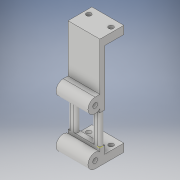
# Autodesk Inventor part: zaxis_clamp2
Saved by Autodesk Inventor 2019 (Build 230136000, 136)
## iProperties
Created: 2020-02-02
Material: Generic
Document SubType Name: Modeling
Designer: Nishant
Density: 1 g/cm^3
Appearance: Default
Author: Nishant
Autodesk Inventor part; units mm, degrees
ref_plane "YZ Plane" through (0, 0, 0) normal (1, 0, 0) x (0, 1, 0)
ref_plane "XZ Plane" through (0, 0, 0) normal (0, 1, 0) x (-1, 0, 0)
ref_plane "XY Plane" through (0, 0, 0) normal (0, 0, 1) x (1, 0, 0)
sketch "Sketch1" plane through (0, 0, 0) normal (1, 0, 0) x (0, 1, 0)
  line L0 (40, 0) -> (40, 3)
  line L1 (40, 3) -> (10, 3)
  line L2 (10, 3) -> (10, 6)
  arc A0 (10, 6) -> (2.1459, 3) centre (5.5, 6) ccw
  line L3 (0, 0) -> (0, 3)
  line L4 (0, 3) -> (2.1459, 3)
  line L5 (40, 0) -> (0, 0)
  circle A1 centre (5.5, 6) radius 1.5
  dimension "d7" = 3
  constraints: 12 end point, 2 centre point, 2 horizontal, 2 point on circle, 2 vertical, 1 coincident, 1 point on line
  measures "d7" diameter of A1
extrude "Extrusion1" add sketch "Sketch1" along normal blind 20
sketch "Sketch2" plane through (0, 0, 0) normal (0, -1, 0) x (1, 0, 0)
  line L0 (0, 0) -> (20, 0) projected
  line L1 (18.5, 0) -> (16.5, 0)
  line L2 (15, 1.5) -> (15, 1.5)
  line L3 (0, 3) -> (20, 3) projected
  line L4 (16.5, 3) -> (18.5, 3)
  line L5 (20, 1.5) -> (20, 1.5)
  arc A0 (20, 1.5) -> (18.5, 3) centre (18.5, 1.5) ccw
  arc A1 (18.5, 0) -> (20, 1.5) centre (18.5, 1.5) ccw
  arc A2 (16.5, 3) -> (15, 1.5) centre (16.5, 1.5) ccw
  arc A3 (15, 1.5) -> (16.5, 0) centre (16.5, 1.5) ccw
  line L6 (0, 6) -> (0, 3) projected
  line L7 (1.5, 3) -> (3.5, 3)
  line L8 (5, 1.5) -> (5, 1.5)
  line L9 (3.5, 0) -> (1.5, 0)
  line L10 (0, 0) -> (0, 3) projected
  line L11 (0, 1.5) -> (0, 1.5)
  arc A4 (5, 1.5) -> (3.5, 3) centre (3.5, 1.5) ccw
  arc A5 (3.5, 0) -> (5, 1.5) centre (3.5, 1.5) ccw
  arc A6 (1.5, 3) -> (0, 1.5) centre (1.5, 1.5) ccw
  arc A7 (0, 1.5) -> (1.5, 0) centre (1.5, 1.5) ccw
  point P0 (15, 0)
  point P1 (15, 3)
  point P2 (5, 3)
  point P3 (5, 0)
  dimension "d10" = 5
  dimension "d11" = 3
  dimension "d12" = 5
  dimension "d13" = 3
  dimension "d14" = 1.5
  dimension "d15" = 5
  dimension "d16" = 3
  dimension "d17" = 5
  dimension "d18" = 3
  dimension "d19" = 1.5
  constraints: 20 point on line, 16 end point, 16 point on circle, 16 tangent, 8 centre point, 6 equal radius, 2 collinear, 2 perpendicular
  measures "d10" distance of L0.end point (15, 0)
  measures "d11" distance of point (15, 0) point (15, 3)
  measures "d12" distance of point (15, 3) L3.end
  measures "d13" distance of L3.end L0.end
  measures "d14" radius of A0
  measures "d15" distance of L3.start point (5, 3)
  measures "d16" distance of point (5, 3) point (5, 0)
  measures "d17" distance of point (5, 0) L0.start
  measures "d18" distance of L0.start L3.start
  measures "d19" radius of A4
extrude "Extrusion2" add sketch "Sketch2" along normal blind 19 contours A7 A6 L3 A4 A5 L0 | A3 A2 L3 A0 A1 L0
ref_plane "Work Plane1" through (18.5, -19, 3) normal (0, -1, 0) x (1, 0, 0)
sketch "Sketch4" plane through (20, 0, 0) normal (1, 0, 0) x (0, 0, -1)
  line L0 (-3, -19) -> (0, -19) projected
  line L1 (0, -19) -> (0, -29)
  line L2 (0, -29) -> (-6, -29)
  arc A0 (-3, -21.1459) -> (-6, -29) centre (-6, -24.5) ccw
  line L3 (-3, -19) -> (-3, -21.1459)
  circle A1 centre (-6, -24.5) radius 1.5
  point P0 (0, 0)
  dimension "d31" = 3
  constraints: 6 end point, 2 centre point, 2 point on circle, 1 coincident, 1 horizontal, 1 vertical
  measures "d31" diameter of A1
extrude "Extrusion3" add sketch "Sketch4" against normal blind 20
sketch "Sketch5" plane through (0, 40, 3) normal (0, 1, 0) x (1, 0, 0)
  line L0 (0, 3) -> (20, 3) projected
  line L1 (20, 3) -> (20, 15)
  line L2 (20, 15) -> (0, 15)
  line L3 (0, 0) -> (0, 3) projected
  line L4 (0, 15) -> (0, 3)
  line L5 (0, 3) -> (20, 3)
  circle A0 centre (17, 10) radius 1.5
  circle A1 centre (3, 10) radius 1.5
  dimension "d34" = 12
  dimension "d35" = 20
  dimension "d36" = 12
  dimension "d37" = 20
  dimension "d40" = 3
  dimension "d43" = 3
  constraints: 8 end point, 2 centre point, 1 perpendicular, 1 vertical
  measures "d34" distance of L0.end L1.end
  measures "d35" distance of L1.end L2.end
  measures "d36" distance of L2.end L0.start
  measures "d37" distance of L0.start L0.end
  measures "d40" diameter of A0
  measures "d43" diameter of A1
extrude "Extrusion4" add sketch "Sketch5" against normal blind 5
sketch "Sketch6" plane through (20, -29, 0) normal (0, -1, 0) x (1, 0, 0)
  line L0 (-20, 0) -> (-20, -12) projected
  line L1 (-20, 0) -> (-20, -12)
  line L2 (-20, -12) -> (0, -12)
  line L3 (-1.5, 0) -> (0, 0) projected
  line L4 (0, -12) -> (0, 0)
  line L5 (0, 0) -> (-20, 0)
  line L6 (-16.5, 0) -> (-3.5, 0) projected
  circle A0 centre (-17, -7) radius 1.5 projected
  circle A1 centre (-17, -7) radius 1.5
  circle A2 centre (-3, -7) radius 1.5 projected
  circle A3 centre (-3, -7) radius 1.5
  dimension "d46" = 12
  dimension "d47" = 20
  dimension "d48" = 12
  dimension "d49" = 20
  dimension "d50" = 3
  dimension "d51" = 3
  constraints: 8 end point, 2 centre point, 2 coincident, 2 collinear, 1 perpendicular
  measures "d46" distance of L0.start L0.end
  measures "d47" distance of L0.end L2.end
  measures "d48" distance of L2.end L3.end
  measures "d49" distance of L3.end L0.start
  measures "d50" diameter of A1
  measures "d51" diameter of A3
extrude "Extrusion5" add sketch "Sketch6" against normal blind 5
body "Solid1"
